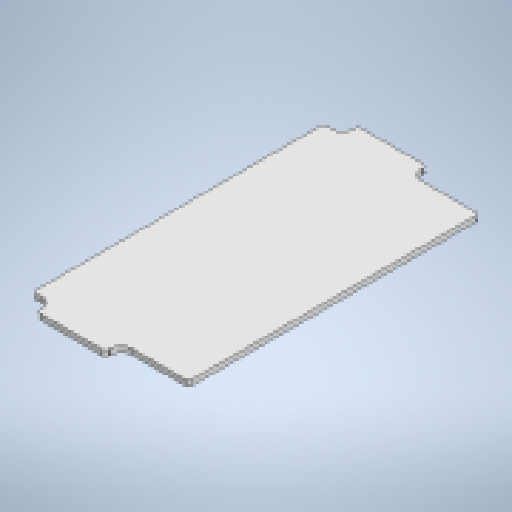
# Autodesk Inventor part: pcb_pre
Saved by Autodesk Inventor 2023 (Build 270158000, 158)
## iProperties
Created: 2025-01-11
Part Number: pcb_pre
Material: Ogólny
Document SubType Name: Modeling
Designer: kamil
Density: 1 g/cm^3
Appearance: Domyślna
Author: kamil
Autodesk Inventor part; units mm, degrees
ref_plane "YZ Plane" through (0, 0, 0) normal (1, 0, 0) x (0, 1, 0)
ref_plane "XZ Plane" through (0, 0, 0) normal (0, 1, 0) x (-1, 0, 0)
ref_plane "XY Plane" through (0, 0, 0) normal (0, 0, 1) x (1, 0, 0)
sketch "Szkic1" plane through (0, 0, 0) normal (0, 1, 0) x (-1, 0, 0)
  line L0 (0, 0) -> (-45, 0)
  line L1 (-45, 0) -> (-45, -84)
  line L2 (-45, -84) -> (0, -84)
  line L3 (0, -84) -> (0, 0)
  dimension "d0" = 45
  dimension "d1" = 84
  constraints: 8 end point, 2 parallel, 1 horizontal, 1 perpendicular
  measures "d0" distance of L2.end L1.end
  measures "d1" distance of L1.end L0.end
extrude "Wyciągnięcie proste1" add sketch "Szkic1" along normal blind 1.6
sketch "Szkic2" plane through (0, 0, 0) normal (0, -1, 0) x (1, 0, 0)
  line L0 (5, 5) -> (5, 4.5) projected
  line L1 (25.8844, 4.5) -> (25.8844, 5) projected
  line L2 (25.8844, -88.5) -> (25.8844, -89) projected
  line L3 (5, -89) -> (5, -88.5) projected
  line L4 (45, 0) -> (45, -84) projected
  line L5 (0, 0) -> (45, 0) projected
  line L6 (0, -84) -> (0, 0) projected
  line L7 (45, -84) -> (0, -84) projected
  line L8 (25.8844, 5) -> (5, 5)
  line L9 (5, 5) -> (5, -3.0099)
  line L10 (5, -3.0099) -> (25.8844, -3.0099)
  line L11 (25.8844, -3.0099) -> (25.8844, 5)
  line L12 (25.8844, -89) -> (5, -89)
  line L13 (5, -89) -> (5, -80.3715)
  line L14 (5, -80.3715) -> (25.8844, -80.3715)
  line L15 (25.8844, -80.3715) -> (25.8844, -89)
  line L16 (25.3844, -88.5) -> (5.5, -88.5)
  line L17 (5.5, -88.5) -> (5.5, -80.8715)
  line L18 (5.5, -80.8715) -> (25.3844, -80.8715)
  line L19 (25.3844, -80.8715) -> (25.3844, -88.5)
  line L20 (25.3844, 4.5) -> (5.5, 4.5)
  line L21 (5.5, 4.5) -> (5.5, -2.5099)
  line L22 (5.5, -2.5099) -> (25.3844, -2.5099)
  line L23 (25.3844, -2.5099) -> (25.3844, 4.5)
  point P0 (25.3844, -84)
  point P1 (5.5, -84)
  point P2 (5.5, 0)
  point P3 (25.3844, 0)
  dimension "d4" = 0.5
  dimension "d5" = 0.5
  constraints: 32 end point, 8 parallel, 4 perpendicular, 2 horizontal, 1 point on line, 6 other
  measures "d4" distance between parallel lines of L15 L19
  measures "d5" distance between parallel lines of L11 L23
extrude "Wyciągnięcie proste2" add sketch "Szkic2" against normal up to surface (1.6 mm away) contours L21 L20 L23 L5 | L7 L19 L16 L17
fillet "Zaokrąglenie1" radius 3 4 edges at (5.5, 0.8, -84) (25.3844, 0.8, -84) (5.5, 0.8, 0) (25.3844, 0.8, 0)
fillet "Zaokrąglenie2" radius 1 8 edges at (25.3844, 0.8, -88.5) (5.5, 0.8, -88.5) (5.5, 0.8, 4.5) (25.3844, 0.8, 4.5) (45, 0.8, 0) (45, 0.8, -84) (0, 0.8, -84) (0, 0.8, 0)
